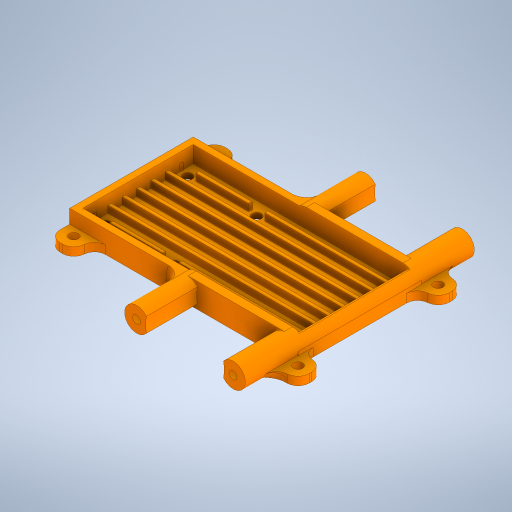
# Autodesk Inventor part: Base
Saved by Autodesk Inventor 2023 (Build 270158000, 158)
## iProperties
Created: 2024-08-05
Part Number: Base
Material: Generic
Document SubType Name: Modeling
Designer: LEGION
Density: 1 g/cm^3
Appearance: Default
Author: LEGION
Autodesk Inventor part; units mm, degrees
ref_plane "YZ Plane" through (0, 0, 0) normal (1, 0, 0) x (0, 1, 0)
ref_plane "XZ Plane" through (0, 0, 0) normal (0, 1, 0) x (-1, 0, 0)
sketch "Sketch1" plane through (0, 0, 0) normal (0, 0, 1) x (1, 0, 0)
  circle A0 centre (0, 0) radius 14.25
  circle A1 centre (-17.5, 0) radius 4.4
  circle A2 centre (17.5, 0) radius 4.4
  circle A3 centre (-17.5, 0) radius 1.4
  circle A4 centre (17.5, 0) radius 1.4
  point P0 (13.9986, -2.6647)
  point P1 (13.9986, 2.6647)
  point P2 (-13.9986, -2.6647)
  point P3 (-13.9986, 2.6647)
  dimension "d0" = 28.5
  dimension "d1" = 17.5
  dimension "d2" = 17.5
  dimension "d3" = 2.8
  dimension "d4" = 2.8
  dimension "d5" = 3
  dimension "d7" = 3
  constraints: 5 centre point, 3 coincident, 2 horizontal alignment
  measures "d0" diameter of A0
  measures "d1" distance of point (0, 0) A2.centre
  measures "d2" distance of point (0, 0) A1.centre
  measures "d3" diameter of A4
  measures "d4" diameter of A3
  measures "d5" radial gap between concentric circles of A1 A3
  measures "d7" radial gap between concentric circles of A4 A2
extrude "Extrusion1" add sketch "Sketch1" along normal blind 18.5 contours A0 A2 | A0 A1 picked at (15.2022, 2.1267) picked at (-14.8909, -1.4953)
sketch "Sketch2" plane through (0, 0, 18.5) normal (0, 0, 1) x (1, 0, 0)
  arc A0 (-13.9986, 2.6647) -> (-13.9986, -2.6647) centre (0, 0) ccw projected
  arc A1 (-13.9986, 2.6647) -> (-13.9986, -2.6647) centre (-17.5, 0) ccw projected
  circle A2 centre (-17.5, 0) radius 1.4 projected
  arc A3 (13.9986, -2.6647) -> (13.9986, 2.6647) centre (0, 0) ccw projected
  arc A4 (13.9986, -2.6647) -> (13.9986, 2.6647) centre (17.5, 0) ccw projected
  circle A5 centre (17.5, 0) radius 1.4 projected
  line L0 (-17.5, 4.4) -> (17.5, 4.4)
  line L1 (17.5, 4.4) -> (17.5, -4.4)
  line L2 (17.5, -4.4) -> (-17.5, -4.4)
  line L3 (-17.5, -4.4) -> (-17.5, 4.4)
  point P0 (-17.5, -4.4)
  dimension "d10" = 4.4
  dimension "d11" = 4.4
  dimension "d12" = 4.4
  dimension "d13" = 0
  dimension "d14" = 0
  constraints: 8 end point, 2 parallel, 1 horizontal, 1 perpendicular
  measures "d10" radius of A4
  measures "d11" distance from line of L0 A4.centre
  measures "d12" distance from line of A4.centre L2
  measures "d13" distance from line of L1 A4.centre
  measures "d14" distance from line of A1.centre L3
extrude "Extrusion2" add sketch "Sketch2" along normal blind 3
ref_plane "Work Plane1" through (0, 0, 41.5) normal (0, 0, 1) x (1, 0, 0)
mirror "Mirror1" about plane through (0, 0, 41.5) normal (0, 0, 1) of "Extrusion1", "Extrusion2"
sketch "Sketch3" plane through (-17.5, -4.4, 18.5) normal (0, -1, 0) x (1, 0, 0)
  line L0 (0, 0) -> (35, 0) projected
  line L1 (35, 0) -> (35, 3) projected
  line L2 (0, 3) -> (35, 3) projected
  line L3 (0, 0) -> (0, 3) projected
  line L4 (0, 46) -> (35, 46) projected
  line L5 (0, 46) -> (0, 43) projected
  line L6 (0, 43) -> (35, 43) projected
  line L7 (35, 46) -> (35, 43) projected
  line L8 (31.4986, -18.5) -> (31.4986, -18.5) projected
  line L9 (31.4986, -18.5) -> (31.4986, 0) projected
  line L10 (35, 0) -> (31.4986, 0) projected
  line L11 (35, 0) -> (35, 3) projected
  line L12 (35, 3) -> (35, 3) projected
  line L13 (35, 0) -> (35, 3) projected
  line L14 (31.4986, 0) -> (35, 0) projected
  line L15 (31.4986, -18.5) -> (31.4986, 0) projected
  line L16 (31.4986, 64.5) -> (31.4986, 64.5) projected
  line L17 (31.4986, 64.5) -> (31.4986, 46) projected
  line L18 (31.4986, 46) -> (35, 46) projected
  line L19 (35, 46) -> (35, 43) projected
  line L20 (35, 43) -> (35, 43) projected
  line L21 (35, 46) -> (35, 43) projected
  line L22 (35, 46) -> (31.4986, 46) projected
  line L23 (31.4986, 64.5) -> (31.4986, 46) projected
  line L24 (39.4, -18.5) -> (39.4, 3) projected
  line L25 (39.4, 43) -> (39.4, 64.5) projected
  line L26 (0, 46) -> (0, 43) projected
  line L27 (0, 45.4) -> (-43.4, 45.4)
  line L28 (-43.4, 45.4) -> (-43.4, 0.6)
  line L29 (-43.4, 0.6) -> (0, 0.6)
  line L30 (0, 0.6) -> (0, 45.4)
  line L31 (35, 45.4) -> (39.4, 45.4)
  line L32 (39.4, 45.4) -> (39.4, 0.6)
  line L33 (39.4, 0.6) -> (35, 0.6)
  line L34 (35, 0.6) -> (35, 45.4)
  point P0 (17.5, -18.5)
  point P1 (0, 0.6)
  dimension "d49" = 2.4
  dimension "d51" = 2.4
  dimension "d52" = 2.4
  dimension "d53" = 2.4
  dimension "d54" = 43.4
  dimension "d56" = 4.4
  constraints: 16 end point, 4 parallel, 2 horizontal, 2 perpendicular, 2 point on line
  measures "d49" distance between parallel lines of L33 L2
  measures "d51" distance between parallel lines of L31 L6
  measures "d52" distance between parallel lines of L29 L2
  measures "d53" distance between parallel lines of L27 L6
  measures "d54" distance between parallel lines of L28 L30
  measures "d56" distance between parallel lines of L34 L32
extrude "Extrusion3" add sketch "Sketch3" against normal blind 2 contours L29 L28 L27 L5 L30 L3 | L30 L6 L34 L2 | L1 L34 L7 L31 L25 L32 L24 L33
sketch "Sketch7" plane through (-17.5, -2.4, 18.5) normal (0, 1, 0) x (1, 0, 0)
  line L0 (38.6878, -3) -> (38.6878, -0.6) projected
  line L1 (-3.6878, -3) -> (38.6878, -3) projected
  line L2 (-3.6878, -0.6) -> (-3.6878, -3) projected
  line L3 (-3.6878, -0.6) -> (-43.4, -0.6) projected
  line L4 (-43.4, -0.6) -> (-43.4, -45.4) projected
  line L5 (-43.4, -45.4) -> (-3.6878, -45.4) projected
  line L6 (-3.6878, -43) -> (-3.6878, -45.4) projected
  line L7 (38.6878, -43) -> (-3.6878, -43) projected
  line L8 (38.6878, -45.4) -> (38.6878, -43) projected
  line L9 (38.6878, -45.4) -> (39.4, -45.4) projected
  line L10 (39.4, -45.4) -> (39.4, -0.6) projected
  line L11 (39.4, -0.6) -> (38.6878, -0.6) projected
  line L12 (39.4, -45.4) -> (35, -45.4) projected
  line L13 (-43.4, -45.4) -> (-43.4, -0.6) projected
  line L14 (39.4, -45.4) -> (-43.4, -45.4)
  line L15 (-43.4, -45.4) -> (-43.4, -0.6)
  line L16 (-43.4, -0.6) -> (39.4, -0.6)
  line L17 (39.4, -0.6) -> (39.4, -45.4)
  line L18 (-41, -43) -> (37, -43)
  line L19 (37, -43) -> (37, -3)
  line L20 (37, -3) -> (-41, -3)
  line L21 (-41, -3) -> (-41, -43)
  point P0 (17.5, 18.5)
  point P1 (37, -3)
  dimension "d57" = 2.4
  constraints: 16 end point, 4 parallel, 2 perpendicular, 1 horizontal, 3 other
  measures "d57" distance between parallel lines of L14 L18
extrude "Extrusion7" add sketch "Sketch7" along normal blind 6 contours L1 L2 L16 L0 | L0 L11 L10 L9 L8 L7 L19 L1 | L2 L20 L21 L18 L6 L5 L4 L3 | L7 L8 L12 L14 L6
sketch "Sketch8" plane through (-17.5, -4.4, 18.5) normal (0, -1, 0) x (1, 0, 0)
  line L0 (42.4, -2.4) -> (-38.88, -2.4)
  line L1 (-38.88, -2.4) -> (-38.88, 48.4)
  line L2 (-38.88, 48.4) -> (42.4, 48.4)
  line L3 (42.4, 48.4) -> (42.4, -2.4)
  line L4 (39.4, 0.6) -> (39.4, 45.4) projected
  circle A0 centre (42.4, -2.4) radius 1.7
  circle A1 centre (-38.88, -2.4) radius 1.7
  line L5 (-43.4, 0.6) -> (0, 0.6) projected
  line L6 (-43.4, 0.6) -> (-34.38, 0.6)
  line L7 (-34.38, 0.6) -> (-34.38, -6.9)
  line L8 (-34.38, -6.9) -> (-43.4, -6.9)
  line L9 (-43.4, -6.9) -> (-43.4, 0.6)
  line L10 (46.9, -6.9) -> (35, -6.9)
  line L11 (35, -6.9) -> (35, 2.1)
  line L12 (35, 2.1) -> (46.9, 2.1)
  line L13 (46.9, 2.1) -> (46.9, -6.9)
  line L14 (35, 0) -> (35, 0.6) projected
  point P0 (17.5, -18.5)
  point P1 (-34.38, -3.15)
  dimension "d60" = 50.8
  dimension "d61" = 81.28
  dimension "d62" = 3
  dimension "d63" = 44.8
  dimension "d64" = 3
  dimension "d65" = 3.4
  dimension "d66" = 3.4
  dimension "d67" = 4.5
  dimension "d68" = 4.5
  dimension "d69" = 4.5
  dimension "d70" = 4.5
  dimension "d71" = 4.5
  constraints: 24 end point, 6 parallel, 3 horizontal, 3 perpendicular, 2 centre point, 2 coincident, 1 collinear, 1 midpoint
  measures "d60" distance of L2.end L0.start
  measures "d61" distance of L0.start L0.end
  measures "d62" distance between parallel lines of L3 L4
  measures "d63" distance of L4.start L4.end
  measures "d64" distance from line of L0 L4.start
  measures "d65" diameter of A0
  measures "d66" diameter of A1
  measures "d67" distance from line of L8 L0.end
  measures "d68" horizontal distance of point (-34.38, -3.15) L0.end
  measures "d69" distance from line of L10 L0.start
  measures "d70" distance from line of L13 L0.start
  measures "d71" distance from line of L0.start L12
extrude "Extrusion8" add sketch "Sketch8" against normal blind 3 contours A1 L1 L5 L7 L0 | L0 L7 L8 L9 L5 L1 A1 | L11 L12 L3 A0 L0 | L0 A0 L3 L12 L13 L10 L11
mirror "Mirror3" about plane through (0, 0, 41.5) normal (0, 0, 1) of "Extrusion8"
fillet "Fillet5" radius 4 8 edges at (29.4, -2.9, 11.6) (29.4, -2.9, 20.6) (-51.88, -2.9, 11.6) (-60.9, -2.9, 11.6) (-60.9, -2.9, 71.4) (-51.88, -2.9, 71.4) (29.4, -2.9, 71.4) (29.4, -2.9, 62.4)
fillet "Fillet6" radius 4 6 edges at (-51.88, -2.9, 19.1) (21.9, -2.9, 20.6) (20.069, -3.5721, 11.6) (21.9, -2.9, 62.4) (20.069, -3.5721, 71.4) (-51.88, -2.9, 63.9)
fillet "Fillet7" radius 4 2 edges at (-21.6952, -1.3266, 63.9) (-21.6952, -1.3266, 19.1)
sketch "Sketch9" plane through (21.9, 3.6, 19.1) normal (0, 0, -1) x (-1, 0, 0)
  arc A0 (1.8702, 0) -> (0, -3.6) centre (4.4, -3.6) ccw projected
  line L0 (0, 0) -> (1.8702, 0) projected
  line L1 (0, -3.6) -> (0, 0) projected
  point P0 (21.9, -3.6)
extrude "Extrusion9" cut sketch "Sketch9" against normal blind 46.75
sketch "Sketch10" plane through (-17.5, -2.4, 18.5) normal (0, 1, 0) x (1, 0, 0)
  line L0 (37, -43) -> (37, -3) projected
  line L1 (37, -3) -> (-41, -3) projected
  line L2 (-41, -3) -> (-41, -43) projected
  line L3 (37, -43) -> (-41, -43) projected
  line L4 (-41, -43) -> (-41, -3) projected
  line L5 (-41, -6.8) -> (37, -6.8)
  line L6 (37, -6.8) -> (37, -8)
  line L7 (37, -8) -> (-41, -8)
  line L8 (-41, -8) -> (-41, -6.8)
  line L9 (-41, -12) -> (37, -12)
  line L10 (37, -12) -> (37, -13.2)
  line L11 (37, -13.2) -> (-41, -13.2)
  line L12 (-41, -13.2) -> (-41, -12)
  line L13 (-41, -17.2) -> (37, -17.2)
  line L14 (37, -17.2) -> (37, -18.4)
  line L15 (37, -18.4) -> (-41, -18.4)
  line L16 (-41, -18.4) -> (-41, -17.2)
  line L17 (-41, -22.4) -> (37, -22.4)
  line L18 (37, -22.4) -> (37, -23.6)
  line L19 (37, -23.6) -> (-41, -23.6)
  line L20 (-41, -23.6) -> (-41, -22.4)
  line L21 (-41, -27.6) -> (37, -27.6)
  line L22 (37, -27.6) -> (37, -28.8)
  line L23 (37, -28.8) -> (-41, -28.8)
  line L24 (-41, -28.8) -> (-41, -27.6)
  line L25 (-41, -32.8) -> (37, -32.8)
  line L26 (37, -32.8) -> (37, -34)
  line L27 (37, -34) -> (-41, -34)
  line L28 (-41, -34) -> (-41, -32.8)
  line L29 (-41, -38) -> (37, -38)
  line L30 (37, -38) -> (37, -39.2)
  line L31 (37, -39.2) -> (-41, -39.2)
  line L32 (-41, -39.2) -> (-41, -38)
  point P0 (17.5, 18.5)
  point P1 (-41, -39.2)
  point P2 (37, -39.2)
  point P3 (-41, -34)
  point P4 (37, -34)
  point P5 (-41, -28.8)
  point P6 (37, -27.6)
  point P7 (-41, -27.6)
  point P8 (-41, -23.6)
  point P9 (37, -23.6)
  point P10 (-41, -18.4)
  point P11 (-41, -13.2)
  point P12 (-41, -8)
  point P13 (37, -6.8)
  dimension "d79" = 3.8
  dimension "d80" = 1.2
  dimension "d81" = 40
  dimension "d84" = 5.2
  dimension "d89" = 3.8
  constraints: 56 end point, 2 parallel, 2 point on line, 1 horizontal, 1 perpendicular, 1 vertical, 48 other
  measures "d79" distance between parallel lines of L1 L5
  measures "d80" distance between parallel lines of L7 L5
  measures "d81" distance of L0.start L0.end
  measures "d84" distance of L5.start L9.start
  measures "d89" distance between parallel lines of L3 L31
extrude "Extrusion10" add sketch "Sketch10" along normal blind 2.5 contours L31 L2 L29 L0 | L27 L2 L25 L0 | L23 L2 L21 L0 | L19 L2 L17 L0 | L15 L2 L13 L0 | L11 L2 L9 L0 | L7 L2 L5 L0
sketch "Sketch11" plane through (-17.5, -4.4, 18.5) normal (0, -1, 0) x (1, 0, 0)
  line L0 (-38, 38) -> (-13, 38)
  line L1 (-13, 38) -> (-13, 8)
  line L2 (-13, 8) -> (-38, 8)
  line L3 (-38, 8) -> (-38, 38)
  line L4 (37, 43) -> (-41, 43) projected
  line L5 (37, 3) -> (-41, 3) projected
  line L6 (-41, 34) -> (-41, 38) projected
  circle A0 centre (-38, 38) radius 1.7
  circle A1 centre (-13, 38) radius 1.7
  circle A2 centre (-13, 8) radius 1.7
  circle A3 centre (-38, 8) radius 1.7
  point P0 (17.5, -18.5)
  dimension "d92" = 30
  dimension "d93" = 25
  dimension "d94" = 5
  dimension "d95" = 40
  dimension "d96" = 3
  dimension "d97" = 3.4
  dimension "d98" = 3.4
  dimension "d99" = 3.4
  dimension "d100" = 3.4
  constraints: 8 end point, 4 centre point, 4 coincident, 2 parallel, 1 horizontal, 1 perpendicular
  measures "d92" distance of L2.end L0.start
  measures "d93" distance of L0.start L0.end
  measures "d94" distance between parallel lines of L4 L0
  measures "d95" distance between parallel lines of L5 L4
  measures "d96" distance between parallel lines of L6 L3
  measures "d97" diameter of A0
  measures "d98" diameter of A1
  measures "d99" diameter of A2
  measures "d100" diameter of A3
extrude "Extrusion11" cut sketch "Sketch11" against normal blind 10 contours L3 A0 L0 | L0 A0 L3 | A1 L1 L0 | L0 L1 A1 | A3 L2 L3 | L3 L2 A3 | A2 L2 L1 | L1 L2 A2
sketch "Sketch12" plane through (-17.5, -2.4, 18.5) normal (0, 1, 0) x (1, 0, 0)
  arc A0 (-14.7, -8) -> (-11.3, -8) centre (-13, -8) ccw projected
  arc A1 (-39.7, -8) -> (-36.3, -8) centre (-38, -8) ccw projected
  arc A2 (-11.3, -38) -> (-14.7, -38) centre (-13, -38) ccw projected
  arc A3 (-36.3, -38) -> (-39.7, -38) centre (-38, -38) ccw projected
  circle A4 centre (-38, -38) radius 3
  circle A5 centre (-13, -38) radius 1.7 projected
  circle A6 centre (-13, -38) radius 3
  circle A7 centre (-13, -8) radius 3
  circle A8 centre (-38, -8) radius 3
  point P0 (17.5, 18.5)
  dimension "d103" = 6
  dimension "d104" = 6
  dimension "d105" = 6
  dimension "d106" = 6
  constraints: 4 centre point, 4 coincident
  measures "d103" diameter of A8
  measures "d104" diameter of A7
  measures "d105" diameter of A6
  measures "d106" diameter of A4
extrude "Extrusion12" cut sketch "Sketch12" along normal blind 10 contours A5 A2 | A4 | A6 | A7 | A8
equation "\"d64\" = 0.5 * d60 - 0.5 * d63"
equation "\"d94\" = 0.5 * d95 - 0.5 * d92"
body "Solid1"
